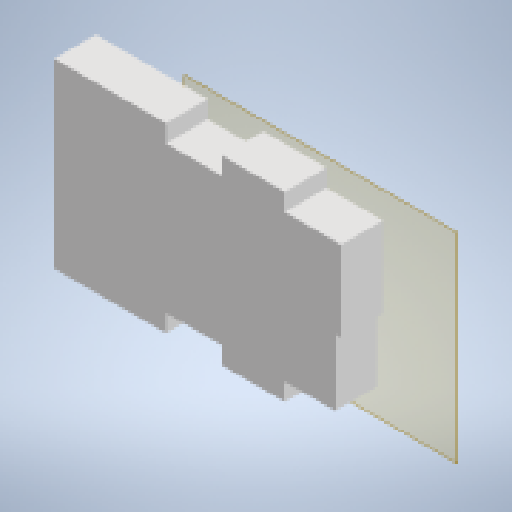
# Autodesk Inventor part: _arm_pit
Saved by Autodesk Inventor 2024.3 (Build 283343000, 343)
## iProperties
Created: 2024-09-06
Part Number: _arm_pit
Material: 일반
Document SubType Name: Modeling
Designer: gretc
Density: 1 g/cm^3
Appearance: 기본값
Author: gretc
Autodesk Inventor part; units mm, degrees
ref_plane "YZ Plane" through (0, 0, 0) normal (1, 0, 0) x (0, 1, 0)
ref_plane "XZ Plane" through (0, 0, 0) normal (0, 1, 0) x (-1, 0, 0)
ref_plane "XY Plane" through (0, 0, 0) normal (0, 0, 1) x (1, 0, 0)
ref_plane "작업 평면1" through (0, 0, 0) normal (0, 0, 1) x (1, 0, 0)
sketch "스케치1" plane through (0, 0, 0) normal (0, 0, 1) x (1, 0, 0)
  line L0 (2, 30.75) -> (2, 4.75) projected
  line L1 (2, 4.75) -> (3.525, 4.75) projected
  line L2 (3.525, 4.75) -> (3.525, 7.25) projected
  line L3 (7.3997, 7.25) -> (3.525, 7.25) projected
  line L4 (7.6003, 7.25) -> (7.3997, 7.25) projected
  line L5 (11.475, 7.25) -> (7.6003, 7.25) projected
  line L6 (11.475, 4.75) -> (11.475, 7.25) projected
  line L7 (11.475, 4.75) -> (20.525, 4.75) projected
  line L8 (20.525, 4.75) -> (20.525, 7.25) projected
  line L9 (24.3997, 7.25) -> (20.525, 7.25) projected
  line L10 (24.6003, 7.25) -> (24.3997, 7.25) projected
  line L11 (27.75, 7.25) -> (24.6003, 7.25) projected
  line L12 (27.75, 16.75) -> (27.75, 7.25) projected
  line L13 (28.6, 16.75) -> (27.75, 16.75) projected
  line L14 (28.6, 16.75) -> (28.6, 28.25) projected
  line L15 (37.525, 28.25) -> (28.6, 28.25) projected
  line L16 (37.525, 30.75) -> (37.525, 28.25) projected
  line L17 (28.475, 30.75) -> (37.525, 30.75) projected
  line L18 (28.475, 30.75) -> (28.475, 28.25) projected
  line L19 (28.475, 28.25) -> (24.6003, 28.25) projected
  line L20 (24.6003, 28.25) -> (24.3997, 28.25) projected
  line L21 (24.3997, 28.25) -> (20.525, 28.25) projected
  line L22 (20.525, 30.75) -> (20.525, 28.25) projected
  line L23 (11.475, 30.75) -> (20.525, 30.75) projected
  line L24 (11.475, 30.75) -> (11.475, 28.25) projected
  line L25 (11.475, 28.25) -> (7.6003, 28.25) projected
  line L26 (7.6003, 28.25) -> (7.3997, 28.25) projected
  line L27 (7.3997, 28.25) -> (3.525, 28.25) projected
  line L28 (3.525, 30.75) -> (3.525, 28.25) projected
  line L29 (2, 30.75) -> (3.525, 30.75) projected
  line L30 (28.6, 28.25) -> (28.475, 28.25)
  line L31 (3.525, 4.75) -> (3.525, 30.75)
  line L32 (3.525, 30.75) -> (-12.475, 30.75)
  line L33 (-12.475, 30.75) -> (-12.475, 4.75)
  line L34 (-12.475, 4.75) -> (3.525, 4.75)
  point P0 (0, 0)
  point P1 (2, 4.75)
  dimension "d0" = 16
  constraints: 10 end point, 2 parallel, 1 horizontal, 1 perpendicular, 1 vertical
  measures "d0" distance of L32.end L28.start
extrude "돌출1" add sketch "스케치1" along normal blind 6 contours L29 L28 L31 L2 L1 L0 | L0 L34 L33 L32 | L27 L26 L25 L24 L23 L22 L21 L20 L19 L30 L14 L13 L12 L11 L10 L9 L8 L7 L6 L5 L4 L3 L31
sketch "스케치2" plane through (20.525, 28.25, 0) normal (0, 1, 0) x (1, 0, 0)
  circle A0 centre (3.975, -2.8) radius 1.35 projected
  circle A1 centre (-13.025, -2.8) radius 1.35 projected
  point P0 (-20.525, 0)
extrude "돌출2" cut sketch "스케치2" against normal up to surface (21 mm away)
sketch "스케치3" plane through (0, 0, 6) normal (0, 0, 1) x (1, 0, 0)
  line L0 (25.85, 28.25) -> (25.85, 7.25) projected
  line L1 (23.15, 28.25) -> (23.15, 7.25) projected
  line L2 (8.85, 28.25) -> (8.85, 7.25) projected
  line L3 (6.15, 28.25) -> (6.15, 7.25) projected
  line L4 (23.15, 7.25) -> (23.15, 13.25)
  line L5 (23.15, 28.25) -> (23.15, 22.25)
  line L6 (23.15, 22.25) -> (6.15, 22.25)
  line L7 (23.15, 22.25) -> (25.85, 22.25)
  line L8 (23.15, 13.25) -> (6.15, 13.25)
  line L9 (23.15, 13.25) -> (25.85, 13.25)
  line L10 (22.5, 14.25) -> (26.5, 14.25)
  line L11 (26.5, 14.25) -> (26.5, 12.25)
  line L12 (26.5, 12.25) -> (22.5, 12.25)
  line L13 (22.5, 12.25) -> (22.5, 14.25)
  line L14 (22.5, 14.25) -> (26.5, 12.25) construction
  line L15 (26.5, 14.25) -> (22.5, 12.25) construction
  line L16 (22.5, 23.25) -> (26.5, 23.25)
  line L17 (26.5, 23.25) -> (26.5, 21.25)
  line L18 (26.5, 21.25) -> (22.5, 21.25)
  line L19 (22.5, 21.25) -> (22.5, 23.25)
  line L20 (22.5, 23.25) -> (26.5, 21.25) construction
  line L21 (26.5, 23.25) -> (22.5, 21.25) construction
  line L22 (6.15, 22.25) -> (7.5, 22.25)
  line L23 (7.5, 22.25) -> (7.5, 13.25)
  line L24 (5.5, 14.25) -> (9.5, 14.25)
  line L25 (9.5, 14.25) -> (9.5, 12.25)
  line L26 (9.5, 12.25) -> (5.5, 12.25)
  line L27 (5.5, 12.25) -> (5.5, 14.25)
  line L28 (5.5, 14.25) -> (9.5, 12.25) construction
  line L29 (9.5, 14.25) -> (5.5, 12.25) construction
  line L30 (5.5, 23.25) -> (9.5, 23.25)
  line L31 (9.5, 23.25) -> (9.5, 21.25)
  line L32 (9.5, 21.25) -> (5.5, 21.25)
  line L33 (5.5, 21.25) -> (5.5, 23.25)
  line L34 (5.5, 23.25) -> (9.5, 21.25) construction
  line L35 (9.5, 23.25) -> (5.5, 21.25) construction
  point P0 (0, 0)
  point P1 (24.5, 13.25)
  point P2 (24.5, 22.25)
  dimension "d5" = 6
  dimension "d6" = 6
  dimension "d7" = 4
  dimension "d8" = 2
  dimension "d9" = 4
  dimension "d10" = 2
  dimension "d11" = 1.35
  dimension "d12" = 4
  dimension "d13" = 2
  dimension "d14" = 4
  dimension "d15" = 2
  constraints: 64 end point, 10 midpoint, 9 point on line, 8 parallel, 8 perpendicular
  measures "d5" distance of L1.end L4.end
  measures "d6" distance of L1.start L5.end
  measures "d7" distance of L10.start L10.end
  measures "d8" distance of L10.end L11.end
  measures "d9" distance of L16.start L16.end
  measures "d10" distance of L16.end L17.end
  measures "d11" distance of L6.end L22.end
  measures "d12" distance of L24.start L24.end
  measures "d13" distance of L24.end L25.end
  measures "d14" distance of L30.start L30.end
  measures "d15" distance of L30.end L31.end
extrude "돌출3" cut sketch "스케치3" against normal blind 6 contours L16 L17 L18 L0 | L0 L7 L1 L16 | L0 L18 L1 L7 | L1 L6 L19 L16 | L1 L18 L19 L6 | L10 L11 L12 L0 | L0 L9 L1 L10 | L0 L12 L1 L9 | L1 L8 L13 L10 | L31 L32 L2 L6 | L6 L2 L30 L31 | L1 L12 L13 L8 | L6 L3 L30 L2 | L2 L32 L23 L6 | L23 L32 L3 L6 | L25 L26 L2 L8 | L8 L2 L24 L25 | L3 L32 L33 L30 | L2 L8 L23 L24 | L2 L26 L3 L8 | L23 L8 L3 L24 | L3 L26 L27 L24
sketch "스케치4" plane through (0, 0, 6) normal (0, 0, 1) x (1, 0, 0)
  line L0 (3.525, 30.75) -> (-12.475, 30.75) projected
  line L1 (-12.475, 30.75) -> (-6.475, 30.75)
  line L2 (-12.475, 4.75) -> (3.525, 4.75) projected
  line L3 (-6.475, 30.75) -> (-0.475, 30.75)
  line L4 (-0.475, 30.75) -> (-0.475, 4.75)
  line L5 (-12.475, 30.75) -> (-12.475, 4.75) projected
  line L6 (-12.475, 30.75) -> (-12.475, 17.75)
  line L7 (-6.475, 30.75) -> (-6.475, 4.75)
  line L8 (-12.475, 17.75) -> (-6.475, 17.75)
  line L9 (-10.975, 20.9166) -> (-10.975, 14.5834)
  line L10 (-10.975, 14.5834) -> (-7.975, 14.5834)
  line L11 (-7.975, 14.5834) -> (-7.975, 20.9166)
  line L12 (-7.975, 20.9166) -> (-10.975, 20.9166)
  line L13 (-10.975, 20.9166) -> (-7.975, 14.5834) construction
  line L14 (-10.975, 14.5834) -> (-7.975, 20.9166) construction
  point P0 (0, 0)
  point P1 (-9.475, 17.75)
  dimension "d18" = 6
  dimension "d19" = 6
  dimension "d22" = 13
  dimension "d23" = 3
  constraints: 24 end point, 5 midpoint, 4 perpendicular, 4 point on line, 2 parallel
  measures "d18" distance of L0.end L1.end
  measures "d19" distance of L1.end L3.end
  measures "d22" distance of L0.end L6.end
  measures "d23" distance of L10.end L9.end
sketch "스케치5" plane through (-12.475, 4.75, 0) normal (-1, 0, 0) x (0, 0, 1)
  line L0 (6, 26) -> (6, 0) projected
  line L1 (0, 0) -> (6, 0) projected
  line L2 (0, 26) -> (0, 0) projected
  line L3 (0, 26) -> (6, 26) projected
  point P0 (0, -4.75)
extrude "돌출4" add sketch "스케치5" along normal blind 6
extrude "돌출5" cut sketch "스케치4" against normal blind 6 contours L11 L10 L9 L8 | L8 L9 L12 L11
sketch "스케치6" plane through (0, 0, 0) normal (0, 0, -1) x (-1, 0, 0)
  point P0 (0, 0)
